Autodesk Fusion 360 part; units mm, degrees
(part 2 of 2)
sketch "Wheel_Hub_PETG_Front_R" plane through (0, 0, 0) normal (1, 0, 0) x (0, 0, -1) in component "Wheel_Hub_PETG_Front_R"
  circle A0 centre (10, 32) radius 22
  line L0 (11.55, 32) -> (11.55, 32.356)
  line L1 (11.55, 32.356) -> (11.55, 32.7011)
  line L2 (11.55, 32.7011) -> (11.55, 33.025)
  line L3 (11.55, 33.025) -> (11.55, 33.3177)
  line L4 (11.55, 33.3177) -> (11.3177, 33.5704)
  line L5 (11.3177, 33.5704) -> (11.025, 33.7754)
  line L6 (11.025, 33.7754) -> (10.7011, 33.9264)
  line L7 (10.7011, 33.9264) -> (10.356, 34.0189)
  line L8 (10.356, 34.0189) -> (10, 34.05)
  line L9 (10, 34.05) -> (9.644, 34.0189)
  line L10 (9.644, 34.0189) -> (9.2989, 33.9264)
  line L11 (9.2989, 33.9264) -> (8.975, 33.7754)
  line L12 (8.975, 33.7754) -> (8.6823, 33.5704)
  line L13 (8.6823, 33.5704) -> (8.4296, 33.3177)
  line L14 (8.4296, 33.3177) -> (8.2246, 33.025)
  line L15 (8.2246, 33.025) -> (8.0736, 32.7011)
  line L16 (8.0736, 32.7011) -> (7.9811, 32.356)
  line L17 (7.9811, 32.356) -> (7.95, 32)
  line L18 (7.95, 32) -> (7.9811, 31.644)
  line L19 (7.9811, 31.644) -> (8.0736, 31.2989)
  line L20 (8.0736, 31.2989) -> (8.2246, 30.975)
  line L21 (8.2246, 30.975) -> (8.4296, 30.6823)
  line L22 (8.4296, 30.6823) -> (8.6823, 30.4296)
  line L23 (8.6823, 30.4296) -> (8.975, 30.2246)
  line L24 (8.975, 30.2246) -> (9.2989, 30.0736)
  line L25 (9.2989, 30.0736) -> (9.644, 29.9811)
  line L26 (9.644, 29.9811) -> (10, 29.95)
  line L27 (10, 29.95) -> (10.356, 29.9811)
  line L28 (10.356, 29.9811) -> (10.7011, 30.0736)
  line L29 (10.7011, 30.0736) -> (11.025, 30.2246)
  line L30 (11.025, 30.2246) -> (11.3177, 30.4296)
  line L31 (11.3177, 30.4296) -> (11.55, 30.6823)
  line L32 (11.55, 30.6823) -> (11.55, 30.975)
  line L33 (11.55, 30.975) -> (11.55, 31.2989)
  line L34 (11.55, 31.2989) -> (11.55, 31.644)
  line L35 (11.55, 31.644) -> (11.55, 32)
extrude "Extrude1''''''''''''''''''''''''''''" add sketch "Wheel_Hub_PETG_Front_R" along normal blind 16 from surface at 62 separate body makes body 29 in component "Wheel_Hub_PETG_Front_R"
sketch "Wheel_Tyre_TPU_Front_R" plane through (0, 0, 0) normal (1, 0, 0) x (0, 0, -1) in component "Wheel_Tyre_TPU_Front_R"
  circle A0 centre (10, 32) radius 32
  circle A1 centre (10, 32) radius 22
extrude "Extrude1'''''''''''''''''''''''''''''" add sketch "Wheel_Tyre_TPU_Front_R" along normal blind 16 from surface at 62 separate body makes body 30 in component "Wheel_Tyre_TPU_Front_R"
sketch "JGA25_370_400rpm_Rear_L" plane through (0, 0, 0) normal (1, 0, 0) x (0, 0, -1) in component "JGA25_370_400rpm_Rear_L"
  circle A0 centre (-70, 32) radius 12.5
extrude "Extrude1''''''''''''''''''''''''''''''" add sketch "JGA25_370_400rpm_Rear_L" along normal blind 52 from surface at -56 separate body makes body 31 in component "JGA25_370_400rpm_Rear_L"
sketch "Wheel_Hub_PETG_Rear_L" plane through (0, 0, 0) normal (1, 0, 0) x (0, 0, -1) in component "Wheel_Hub_PETG_Rear_L"
  circle A0 centre (-70, 32) radius 22
  line L0 (-68.45, 32) -> (-68.45, 32.356)
  line L1 (-68.45, 32.356) -> (-68.45, 32.7011)
  line L2 (-68.45, 32.7011) -> (-68.45, 33.025)
  line L3 (-68.45, 33.025) -> (-68.45, 33.3177)
  line L4 (-68.45, 33.3177) -> (-68.6823, 33.5704)
  line L5 (-68.6823, 33.5704) -> (-68.975, 33.7754)
  line L6 (-68.975, 33.7754) -> (-69.2989, 33.9264)
  line L7 (-69.2989, 33.9264) -> (-69.644, 34.0189)
  line L8 (-69.644, 34.0189) -> (-70, 34.05)
  line L9 (-70, 34.05) -> (-70.356, 34.0189)
  line L10 (-70.356, 34.0189) -> (-70.7011, 33.9264)
  line L11 (-70.7011, 33.9264) -> (-71.025, 33.7754)
  line L12 (-71.025, 33.7754) -> (-71.3177, 33.5704)
  line L13 (-71.3177, 33.5704) -> (-71.5704, 33.3177)
  line L14 (-71.5704, 33.3177) -> (-71.7754, 33.025)
  line L15 (-71.7754, 33.025) -> (-71.9264, 32.7011)
  line L16 (-71.9264, 32.7011) -> (-72.0189, 32.356)
  line L17 (-72.0189, 32.356) -> (-72.05, 32)
  line L18 (-72.05, 32) -> (-72.0189, 31.644)
  line L19 (-72.0189, 31.644) -> (-71.9264, 31.2989)
  line L20 (-71.9264, 31.2989) -> (-71.7754, 30.975)
  line L21 (-71.7754, 30.975) -> (-71.5704, 30.6823)
  line L22 (-71.5704, 30.6823) -> (-71.3177, 30.4296)
  line L23 (-71.3177, 30.4296) -> (-71.025, 30.2246)
  line L24 (-71.025, 30.2246) -> (-70.7011, 30.0736)
  line L25 (-70.7011, 30.0736) -> (-70.356, 29.9811)
  line L26 (-70.356, 29.9811) -> (-70, 29.95)
  line L27 (-70, 29.95) -> (-69.644, 29.9811)
  line L28 (-69.644, 29.9811) -> (-69.2989, 30.0736)
  line L29 (-69.2989, 30.0736) -> (-68.975, 30.2246)
  line L30 (-68.975, 30.2246) -> (-68.6823, 30.4296)
  line L31 (-68.6823, 30.4296) -> (-68.45, 30.6823)
  line L32 (-68.45, 30.6823) -> (-68.45, 30.975)
  line L33 (-68.45, 30.975) -> (-68.45, 31.2989)
  line L34 (-68.45, 31.2989) -> (-68.45, 31.644)
  line L35 (-68.45, 31.644) -> (-68.45, 32)
extrude "Extrude1'''''''''''''''''''''''''''''''" add sketch "Wheel_Hub_PETG_Rear_L" along normal blind 16 from surface at -78 separate body makes body 32 in component "Wheel_Hub_PETG_Rear_L"
sketch "Wheel_Tyre_TPU_Rear_L" plane through (0, 0, 0) normal (1, 0, 0) x (0, 0, -1) in component "Wheel_Tyre_TPU_Rear_L"
  circle A0 centre (-70, 32) radius 32
  circle A1 centre (-70, 32) radius 22
extrude "Extrude1''''''''''''''''''''''''''''''''" add sketch "Wheel_Tyre_TPU_Rear_L" along normal blind 16 from surface at -78 separate body makes body 33 in component "Wheel_Tyre_TPU_Rear_L"
sketch "JGA25_370_400rpm_Rear_R" plane through (0, 0, 0) normal (1, 0, 0) x (0, 0, -1) in component "JGA25_370_400rpm_Rear_R"
  circle A0 centre (-70, 32) radius 12.5
extrude "Extrude1'''''''''''''''''''''''''''''''''" add sketch "JGA25_370_400rpm_Rear_R" along normal blind 52 from surface at 4 separate body makes body 34 in component "JGA25_370_400rpm_Rear_R"
sketch "Wheel_Hub_PETG_Rear_R" plane through (0, 0, 0) normal (1, 0, 0) x (0, 0, -1) in component "Wheel_Hub_PETG_Rear_R"
  circle A0 centre (-70, 32) radius 22
  line L0 (-68.45, 32) -> (-68.45, 32.356)
  line L1 (-68.45, 32.356) -> (-68.45, 32.7011)
  line L2 (-68.45, 32.7011) -> (-68.45, 33.025)
  line L3 (-68.45, 33.025) -> (-68.45, 33.3177)
  line L4 (-68.45, 33.3177) -> (-68.6823, 33.5704)
  line L5 (-68.6823, 33.5704) -> (-68.975, 33.7754)
  line L6 (-68.975, 33.7754) -> (-69.2989, 33.9264)
  line L7 (-69.2989, 33.9264) -> (-69.644, 34.0189)
  line L8 (-69.644, 34.0189) -> (-70, 34.05)
  line L9 (-70, 34.05) -> (-70.356, 34.0189)
  line L10 (-70.356, 34.0189) -> (-70.7011, 33.9264)
  line L11 (-70.7011, 33.9264) -> (-71.025, 33.7754)
  line L12 (-71.025, 33.7754) -> (-71.3177, 33.5704)
  line L13 (-71.3177, 33.5704) -> (-71.5704, 33.3177)
  line L14 (-71.5704, 33.3177) -> (-71.7754, 33.025)
  line L15 (-71.7754, 33.025) -> (-71.9264, 32.7011)
  line L16 (-71.9264, 32.7011) -> (-72.0189, 32.356)
  line L17 (-72.0189, 32.356) -> (-72.05, 32)
  line L18 (-72.05, 32) -> (-72.0189, 31.644)
  line L19 (-72.0189, 31.644) -> (-71.9264, 31.2989)
  line L20 (-71.9264, 31.2989) -> (-71.7754, 30.975)
  line L21 (-71.7754, 30.975) -> (-71.5704, 30.6823)
  line L22 (-71.5704, 30.6823) -> (-71.3177, 30.4296)
  line L23 (-71.3177, 30.4296) -> (-71.025, 30.2246)
  line L24 (-71.025, 30.2246) -> (-70.7011, 30.0736)
  line L25 (-70.7011, 30.0736) -> (-70.356, 29.9811)
  line L26 (-70.356, 29.9811) -> (-70, 29.95)
  line L27 (-70, 29.95) -> (-69.644, 29.9811)
  line L28 (-69.644, 29.9811) -> (-69.2989, 30.0736)
  line L29 (-69.2989, 30.0736) -> (-68.975, 30.2246)
  line L30 (-68.975, 30.2246) -> (-68.6823, 30.4296)
  line L31 (-68.6823, 30.4296) -> (-68.45, 30.6823)
  line L32 (-68.45, 30.6823) -> (-68.45, 30.975)
  line L33 (-68.45, 30.975) -> (-68.45, 31.2989)
  line L34 (-68.45, 31.2989) -> (-68.45, 31.644)
  line L35 (-68.45, 31.644) -> (-68.45, 32)
extrude "Extrude1''''''''''''''''''''''''''''''''''" add sketch "Wheel_Hub_PETG_Rear_R" along normal blind 16 from surface at 62 separate body makes body 35 in component "Wheel_Hub_PETG_Rear_R"
sketch "Wheel_Tyre_TPU_Rear_R" plane through (0, 0, 0) normal (1, 0, 0) x (0, 0, -1) in component "Wheel_Tyre_TPU_Rear_R"
  circle A0 centre (-70, 32) radius 32
  circle A1 centre (-70, 32) radius 22
extrude "Extrude1'''''''''''''''''''''''''''''''''''" add sketch "Wheel_Tyre_TPU_Rear_R" along normal blind 16 from surface at 62 separate body makes body 36 in component "Wheel_Tyre_TPU_Rear_R"
sketch "Sketch1 (8)" plane through (0, 0, 0) normal (0, 1, 0) x (1, 0, 0) in component "3S_850mAh_LiPo_ENVELOPE_75x35x25"
  line L0 (-37.5, -38) -> (37.5, -38)
  line L1 (37.5, -38) -> (37.5, -3)
  line L2 (37.5, -3) -> (-37.5, -3)
  line L3 (-37.5, -3) -> (-37.5, -38)
extrude "Extrude1''''''''''''''''''''''''''''''''''''" add sketch "Sketch1 (8)" along normal blind 25 from surface at 8 separate body makes body 37 in component "3S_850mAh_LiPo_ENVELOPE_75x35x25"
sketch "Sketch1 (9)" plane through (0, 0, 0) normal (0, 1, 0) x (1, 0, 0) in component "Skywalker_40A_ESC_55x25x12"
  line L0 (-60, -40) -> (-5, -40)
  line L1 (-5, -40) -> (-5, -15)
  line L2 (-5, -15) -> (-60, -15)
  line L3 (-60, -15) -> (-60, -40)
extrude "Extrude1'''''''''''''''''''''''''''''''''''''" add sketch "Sketch1 (9)" along normal blind 12 from surface at 34 separate body makes body 38 in component "Skywalker_40A_ESC_55x25x12"
sketch "Sketch1 (10)" plane through (0, 0, 0) normal (0, 1, 0) x (1, 0, 0) in component "ESP32_DevKit_51.5x28.3"
  line L0 (4, -42) -> (55.5, -42)
  line L1 (55.5, -42) -> (55.5, -13.7)
  line L2 (55.5, -13.7) -> (4, -13.7)
  line L3 (4, -13.7) -> (4, -42)
extrude "Extrude1''''''''''''''''''''''''''''''''''''''" add sketch "Sketch1 (10)" along normal blind 14 from surface at 34 separate body makes body 39 in component "ESP32_DevKit_51.5x28.3"
sketch "Sketch1 (11)" plane through (0, 0, 0) normal (0, 1, 0) x (1, 0, 0) in component "DRV8871_L"
  line L0 (39, -45) -> (59, -45)
  line L1 (59, -45) -> (59, -25)
  line L2 (59, -25) -> (39, -25)
  line L3 (39, -25) -> (39, -45)
extrude "Extrude1'''''''''''''''''''''''''''''''''''''''" add sketch "Sketch1 (11)" along normal blind 6 from surface at 8 separate body makes body 40 in component "DRV8871_L"
sketch "Sketch1 (12)" plane through (0, 0, 0) normal (0, 1, 0) x (1, 0, 0) in component "DRV8871_R"
  line L0 (39, -24) -> (59, -24)
  line L1 (59, -24) -> (59, -4)
  line L2 (59, -4) -> (39, -4)
  line L3 (39, -4) -> (39, -24)
extrude "Extrude1''''''''''''''''''''''''''''''''''''''''" add sketch "Sketch1 (12)" along normal blind 6 from surface at 8 separate body makes body 41 in component "DRV8871_R"
sketch "Sketch1 (13)" plane through (0, 0, 0) normal (0, 1, 0) x (1, 0, 0) in component "IMU_Foam_Pad_1mm"
  line L0 (-10.5, -56) -> (10.5, -56)
  line L1 (10.5, -56) -> (10.5, -40)
  line L2 (10.5, -40) -> (-10.5, -40)
  line L3 (-10.5, -40) -> (-10.5, -56)
extrude "Extrude1'''''''''''''''''''''''''''''''''''''''''" add sketch "Sketch1 (13)" along normal blind 1 from surface at 7 separate body makes body 42 in component "IMU_Foam_Pad_1mm"
sketch "Sketch1 (14)" plane through (0, 0, 0) normal (0, 1, 0) x (1, 0, 0) in component "IMU_GY521_MPU6050_21x16"
  line L0 (-10.5, -56) -> (10.5, -56)
  line L1 (10.5, -56) -> (10.5, -40)
  line L2 (10.5, -40) -> (-10.5, -40)
  line L3 (-10.5, -40) -> (-10.5, -56)
extrude "Extrude1''''''''''''''''''''''''''''''''''''''''''" add sketch "Sketch1 (14)" along normal blind 3.5 from surface at 8 separate body makes body 43 in component "IMU_GY521_MPU6050_21x16"
sketch "Sketch1 (15)" plane through (0, 0, 0) normal (0, 1, 0) x (1, 0, 0) in component "Hall_Post_PETG"
  line L0 (8, 40) -> (12, 40)
  line L1 (12, 40) -> (12, 48)
  line L2 (12, 48) -> (8, 48)
  line L3 (8, 48) -> (8, 40)
extrude "Extrude1'''''''''''''''''''''''''''''''''''''''''''" add sketch "Sketch1 (15)" along normal blind 36 from surface at 7 separate body makes body 44 in component "Hall_Post_PETG"
sketch "Sketch1 (16)" plane through (0, 0, 0) normal (0, 1, 0) x (1, 0, 0) in component "Hall_A3144_TO92"
  line L0 (6.5, 42) -> (8, 42)
  line L1 (8, 42) -> (8, 46)
  line L2 (8, 46) -> (6.5, 46)
  line L3 (6.5, 46) -> (6.5, 42)
extrude "Extrude1''''''''''''''''''''''''''''''''''''''''''''" add sketch "Sketch1 (16)" along normal blind 4 from surface at 37 separate body makes body 45 in component "Hall_A3144_TO92"
sketch "Sketch1 (17)" plane through (0, 0, 0) normal (0, 1, 0) x (1, 0, 0) in component "Power_Switch_Link"
  line L0 (66, -34) -> (80, -34)
  line L1 (80, -34) -> (80, -26)
  line L2 (80, -26) -> (66, -26)
  line L3 (66, -26) -> (66, -34)
extrude "Extrude1'''''''''''''''''''''''''''''''''''''''''''''" add sketch "Sketch1 (17)" along normal blind 10 from surface at 20 separate body makes body 46 in component "Power_Switch_Link"
component "01_Printed_Chassis_TPU" placed x (1, 0, 0) y (0, 1, 0) z (0, 0, 1) at (0, 0, 0)
component "02_Weapon_Beater" placed x (1, 0, 0) y (0, 1, 0) z (0, 0, 1) at (0, 0, 0)
component "03_Steel_Wedgelets_2mm" placed x (1, 0, 0) y (0, 1, 0) z (0, 0, 1) at (0, 0, 0)
component "04_Drive_4WD" placed x (1, 0, 0) y (0, 1, 0) z (0, 0, 1) at (0, 0, 0)
component "05_Electronics_ENVELOPES" placed x (1, 0, 0) y (0, 1, 0) z (0, 0, 1) at (0, 0, 0)
component "Tub_TPU" placed x (1, 0, 0) y (0, 1, 0) z (0, 0, 1) at (0, 0, 0) in component "01_Printed_Chassis_TPU"
component "Lid_TPU_3mm" placed x (1, 0, 0) y (0, 1, 0) z (0, 0, 1) at (0, 0, 0) in component "01_Printed_Chassis_TPU"
component "Upright_6061_6mm_L" placed x (1, 0, 0) y (0, 1, 0) z (0, 0, 1) at (0, 0, 0) in component "02_Weapon_Beater"
component "Upright_6061_6mm_R" placed x (1, 0, 0) y (0, 1, 0) z (0, 0, 1) at (0, 0, 0) in component "02_Weapon_Beater"
component "Weapon_Top_Brace_3mm" placed x (1, 0, 0) y (0, 1, 0) z (0, 0, 1) at (0, 0, 0) in component "02_Weapon_Beater"
component "Weapon_Bottom_Brace_3mm" placed x (1, 0, 0) y (0, 1, 0) z (0, 0, 1) at (0, 0, 0) in component "02_Weapon_Beater"
component "Beater_Disc_L" placed x (1, 0, 0) y (0, 1, 0) z (0, 0, 1) at (0, 0, 0) in component "02_Weapon_Beater"
component "Beater_Disc_R" placed x (1, 0, 0) y (0, 1, 0) z (0, 0, 1) at (0, 0, 0) in component "02_Weapon_Beater"
component "Beater_Hub_6061_D30" placed x (1, 0, 0) y (0, 1, 0) z (0, 0, 1) at (0, 0, 0) in component "02_Weapon_Beater"
component "Bearing_608_L" placed x (1, 0, 0) y (0, 1, 0) z (0, 0, 1) at (0, 0, 0) in component "02_Weapon_Beater"
component "Bearing_608_R" placed x (1, 0, 0) y (0, 1, 0) z (0, 0, 1) at (0, 0, 0) in component "02_Weapon_Beater"
component "Spacer_Outer_L_ID8.2_OD11" placed x (1, 0, 0) y (0, 1, 0) z (0, 0, 1) at (0, 0, 0) in component "02_Weapon_Beater"
component "Spacer_Inner_ID8.2_OD11" placed x (1, 0, 0) y (0, 1, 0) z (0, 0, 1) at (0, 0, 0) in component "02_Weapon_Beater"
component "Spacer_Outer_R_ID8.2_OD11" placed x (1, 0, 0) y (0, 1, 0) z (0, 0, 1) at (0, 0, 0) in component "02_Weapon_Beater"
component "Dead_Shaft_M8_12.9" placed x (1, 0, 0) y (0, 1, 0) z (0, 0, 1) at (0, 0, 0) in component "02_Weapon_Beater"
component "D3536_1250kV_Can_ENVELOPE" placed x (1, 0, 0) y (0, 1, 0) z (0, 0, 1) at (0, 0, 0) in component "02_Weapon_Beater"
component "Motor_Pulley_D26_Groove" placed x (1, 0, 0) y (0, 1, 0) z (0, 0, 1) at (0, 0, 0) in component "02_Weapon_Beater"
component "Weapon_Motor_Mount_3mm" placed x (1, 0, 0) y (0, 1, 0) z (0, 0, 1) at (0, 0, 0) in component "02_Weapon_Beater"
component "Belt_Upper_ENVELOPE" placed x (1, 0, 0) y (0, 1, 0) z (0, 0, 1) at (0, 0, 0) in component "02_Weapon_Beater"
component "Belt_Lower_ENVELOPE" placed x (1, 0, 0) y (0, 1, 0) z (0, 0, 1) at (0, 0, 0) in component "02_Weapon_Beater"
component "Wedgelet_L" placed x (1, 0, 0) y (0, 1, 0) z (0, 0, 1) at (0, 0, 0) in component "03_Steel_Wedgelets_2mm"
component "Wedgelet_R" placed x (1, 0, 0) y (0, 1, 0) z (0, 0, 1) at (0, 0, 0) in component "03_Steel_Wedgelets_2mm"
component "Wedgelet_Block_PETG_L" placed x (1, 0, 0) y (0, 1, 0) z (0, 0, 1) at (0, 0, 0) in component "03_Steel_Wedgelets_2mm"
component "Wedgelet_Block_PETG_R" placed x (1, 0, 0) y (0, 1, 0) z (0, 0, 1) at (0, 0, 0) in component "03_Steel_Wedgelets_2mm"
component "01_Printed_Chassis_TPU" placed x (1, 0, 0) y (0, 1, 0) z (0, 0, 1) at (0, 0, 0) in component "Wedgelet_L"
component "JGA25_370_400rpm_Front_L" placed x (1, 0, 0) y (0, 1, 0) z (0, 0, 1) at (0, 0, 0) in component "04_Drive_4WD"
component "Wheel_Hub_PETG_Front_L" placed x (1, 0, 0) y (0, 1, 0) z (0, 0, 1) at (0, 0, 0) in component "04_Drive_4WD"
component "Wheel_Tyre_TPU_Front_L" placed x (1, 0, 0) y (0, 1, 0) z (0, 0, 1) at (0, 0, 0) in component "04_Drive_4WD"
component "JGA25_370_400rpm_Front_R" placed x (1, 0, 0) y (0, 1, 0) z (0, 0, 1) at (0, 0, 0) in component "04_Drive_4WD"
component "Wheel_Hub_PETG_Front_R" placed x (1, 0, 0) y (0, 1, 0) z (0, 0, 1) at (0, 0, 0) in component "04_Drive_4WD"
component "Wheel_Tyre_TPU_Front_R" placed x (1, 0, 0) y (0, 1, 0) z (0, 0, 1) at (0, 0, 0) in component "04_Drive_4WD"
component "JGA25_370_400rpm_Rear_L" placed x (1, 0, 0) y (0, 1, 0) z (0, 0, 1) at (0, 0, 0) in component "04_Drive_4WD"
component "Wheel_Hub_PETG_Rear_L" placed x (1, 0, 0) y (0, 1, 0) z (0, 0, 1) at (0, 0, 0) in component "04_Drive_4WD"
component "Wheel_Tyre_TPU_Rear_L" placed x (1, 0, 0) y (0, 1, 0) z (0, 0, 1) at (0, 0, 0) in component "04_Drive_4WD"
component "JGA25_370_400rpm_Rear_R" placed x (1, 0, 0) y (0, 1, 0) z (0, 0, 1) at (0, 0, 0) in component "04_Drive_4WD"
component "Wheel_Hub_PETG_Rear_R" placed x (1, 0, 0) y (0, 1, 0) z (0, 0, 1) at (0, 0, 0) in component "04_Drive_4WD"
component "Wheel_Tyre_TPU_Rear_R" placed x (1, 0, 0) y (0, 1, 0) z (0, 0, 1) at (0, 0, 0) in component "04_Drive_4WD"
component "Tub_TPU" placed x (1, 0, 0) y (0, 1, 0) z (0, 0, 1) at (0, 0, 0) in component "Wheel_Tyre_TPU_Front_L"
component "3S_850mAh_LiPo_ENVELOPE_75x35x25" placed x (1, 0, 0) y (0, 1, 0) z (0, 0, 1) at (0, 0, 0) in component "05_Electronics_ENVELOPES"
component "Skywalker_40A_ESC_55x25x12" placed x (1, 0, 0) y (0, 1, 0) z (0, 0, 1) at (0, 0, 0) in component "05_Electronics_ENVELOPES"
component "ESP32_DevKit_51.5x28.3" placed x (1, 0, 0) y (0, 1, 0) z (0, 0, 1) at (0, 0, 0) in component "05_Electronics_ENVELOPES"
component "DRV8871_L" placed x (1, 0, 0) y (0, 1, 0) z (0, 0, 1) at (0, 0, 0) in component "05_Electronics_ENVELOPES"
component "DRV8871_R" placed x (1, 0, 0) y (0, 1, 0) z (0, 0, 1) at (0, 0, 0) in component "05_Electronics_ENVELOPES"
component "IMU_Foam_Pad_1mm" placed x (1, 0, 0) y (0, 1, 0) z (0, 0, 1) at (0, 0, 0) in component "05_Electronics_ENVELOPES"
component "IMU_GY521_MPU6050_21x16" placed x (1, 0, 0) y (0, 1, 0) z (0, 0, 1) at (0, 0, 0) in component "05_Electronics_ENVELOPES"
component "Hall_Post_PETG" placed x (1, 0, 0) y (0, 1, 0) z (0, 0, 1) at (0, 0, 0) in component "05_Electronics_ENVELOPES"
component "Hall_A3144_TO92" placed x (1, 0, 0) y (0, 1, 0) z (0, 0, 1) at (0, 0, 0) in component "05_Electronics_ENVELOPES"
component "Power_Switch_Link" placed x (1, 0, 0) y (0, 1, 0) z (0, 0, 1) at (0, 0, 0) in component "05_Electronics_ENVELOPES"
named bodies: "Tub_TPU", "Lid_TPU_3mm", "Upright_6061_6mm_L", "Upright_6061_6mm_R", "Weapon_Top_Brace_3mm", "Weapon_Bottom_Brace_3mm", "Beater_Disc_L", "Beater_Disc_R", "Beater_Hub_6061_D30", "Bearing_608_L", "Bearing_608_R", "Spacer_Outer_L_ID8.2_OD11", "Spacer_Inner_ID8.2_OD11", "Spacer_Outer_R_ID8.2_OD11", "Dead_Shaft_M8_12.9", "D3536_1250kV_Can_ENVELOPE", "Motor_Pulley_D26_Groove", "Weapon_Motor_Mount_3mm", "Belt_Upper_ENVELOPE", "Belt_Lower_ENVELOPE", "Wedgelet_L", "Wedgelet_R", "Wedgelet_Block_PETG_L", "Wedgelet_Block_PETG_R", "JGA25_370_400rpm_Front_L", "Wheel_Hub_PETG_Front_L", "Wheel_Tyre_TPU_Front_L", "JGA25_370_400rpm_Front_R", "Wheel_Hub_PETG_Front_R", "Wheel_Tyre_TPU_Front_R", "JGA25_370_400rpm_Rear_L", "Wheel_Hub_PETG_Rear_L", "Wheel_Tyre_TPU_Rear_L", "JGA25_370_400rpm_Rear_R", "Wheel_Hub_PETG_Rear_R", "Wheel_Tyre_TPU_Rear_R", "3S_850mAh_LiPo_ENVELOPE_75x35x25", "Skywalker_40A_ESC_55x25x12", "ESP32_DevKit_51.5x28.3", "DRV8871_L", "DRV8871_R", "IMU_Foam_Pad_1mm", "IMU_GY521_MPU6050_21x16", "Hall_Post_PETG", "Hall_A3144_TO92", "Power_Switch_Link"
